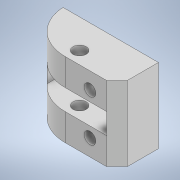
# Autodesk Inventor part: Abzughalter
Saved by Autodesk Inventor 2021 (Build 250183000, 183)
## iProperties
Created: 2024-05-16
Part Number: Abzughalter
Material: Generic
Document SubType Name: Modeling
Designer: Lukas
Density: 1 g/cm^3
Appearance: Default
Author: Lukas
Autodesk Inventor part; units mm, degrees
ref_plane "YZ Plane" through (0, 0, 0) normal (1, 0, 0) x (0, 1, 0)
ref_plane "XZ Plane" through (0, 0, 0) normal (0, 1, 0) x (-1, 0, 0)
ref_plane "XY Plane" through (0, 0, 0) normal (0, 0, 1) x (1, 0, 0)
sketch "Sketch1" plane through (0, 0, 0) normal (0, 0, 1) x (1, 0, 0)
  line L0 (-9, 2.5) -> (9, 2.5)
  line L1 (9, 2.5) -> (9, -2.5)
  line L2 (9, -2.5) -> (-9, -2.5)
  line L3 (-9, -2.5) -> (-9, 2.5)
  line L4 (-11.5, 9) -> (11.5, 9)
  line L5 (11.5, 9) -> (11.5, -9)
  line L6 (11.5, -9) -> (-11.5, -9)
  line L7 (-11.5, -9) -> (-11.5, 9)
  circle A0 centre (5, 5) radius 1.4
  circle A1 centre (5, -5) radius 1.4
  point P0 (0, 0)
  point P1 (0, 2.5)
  point P2 (-9, 0)
  point P3 (-11.5, 0)
  dimension "d0" = 5
  dimension "d1" = 5
  dimension "d2" = 5
  dimension "d3" = 18
  dimension "d5" = 4
  dimension "d6" = 2.8
  dimension "d7" = 2.5
  dimension "d8" = 2.5
  dimension "d9" = 18
  constraints: 16 end point, 4 parallel, 3 midpoint, 2 centre point, 2 horizontal, 2 horizontal alignment, 2 perpendicular, 2 vertical alignment, 1 equal radius
  measures "d0" horizontal distance of A0.centre point (0, 0)
  measures "d1" horizontal distance of point (0, 0) A1.centre
  measures "d2" distance of L0.end L1.end
  measures "d3" distance of L0.start L0.end
  measures "d5" distance from line of L1 A0.centre
  measures "d6" diameter of A0
  measures "d7" distance between parallel lines of L7 L3
  measures "d8" distance between parallel lines of L5 L1
  measures "d9" distance of L4.end L5.end
extrude "Extrusion1" add sketch "Sketch1" along normal blind 10
sketch "Sketch2" plane through (-11.5, 9, 0) normal (0, 1, 0) x (1, 0, 0)
  circle A0 centre (11, -7) radius 1.6
  line L0 (23, -10) -> (0, -10) projected
  line L1 (0, 0) -> (0, -10) projected
  point P0 (11.5, 0)
  dimension "d12" = 3
  dimension "d13" = 3.2
  dimension "d14" = 11
  constraints: 1 centre point
  measures "d12" distance from line of L0 A0.centre
  measures "d13" diameter of A0
  measures "d14" distance from line of L1 A0.centre
extrude "Extrusion2" cut sketch "Sketch2" against normal through all
chamfer "Chamfer1" distance 6 angle 45 1 edges at (-11.5, 0, 10)
chamfer "Chamfer2" distance 2.5 angle 45 1 edges at (11.5, 0, 10)
fillet "Fillet1" radius 10.5 3 edges at (-5.5, 5.75, 10) (-5.5, -5.75, 10) (-11.5, 0, 4)
equation "\"d1\" = d0"
equation "\"d7\" = d8"
body "Solid1"
